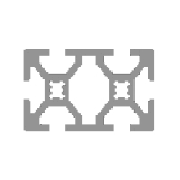
# Autodesk Inventor part: 20-2040
Saved by Autodesk Inventor 2021 (Build 250183000, 183)
## iProperties
IsCustomPart: 1
_CCFamilyDisplayName: 20-2040
_FrameMemberDoc: Frame Member File
_Version: 15.0.0
_GetPNFromCC: 1
Created: 2020-11-09
Part Number: 20-2040
Material: Generic
Document SubType Name: Modeling
Designer: Wes
Manufacturer: 8020
Standards Organization: 8020 Metric
Language: en-US
Size Designation: 20-2040
Categories: <MemberInstance><Categories><Category DisplayName="Structural Shapes" InternalName="089c4875-fa83-4c05-b084-43b9cc11f5ed" Mnemonic="GRDR"><CategoryParameter DisplayName="Mass per Length Unit" InternalName="0bb95a10-148f-4027-a459-38d7b056702a" Mnemonic="shpmass"/><CategoryParameter DisplayName="Section Area" InternalName="1ff91680-64b0-4202-b9a3-7fd3f94bba3b" Mnemonic="secarea"/><CategoryParameter DisplayName="Radius of Gyration (x)" InternalName="25778675-03e9-40c1-b6a8-4a9ed693320d" Mnemonic="gyrradx"/><CategoryParameter DisplayName="Torsional Rigidity Modulus" InternalName="26c1ec35-5026-4c63-ad0a-751cf684a536" Mnemonic="torrigmod"/><CategoryParameter DisplayName="Distance of the Center of Gravity X-X" InternalName="26c9bdb8-9c79-4b4f-a92e-8e197583c9c4" Mnemonic="grcendistX"/><CategoryParameter DisplayName="Legacy Member ID" InternalName="340afe4f-75d7-48d3-ab7d-943f3c3da468" Mnemonic="LegacyMemberID"/><CategoryParameter DisplayName="Base Length" InternalName="42e34263-8f20-4d0e-ad48-bf1385b87c24" Mnemonic="shplen"/><CategoryParameter DisplayName="Moment of Inertia (y)" InternalName="4b9f58ea-bced-460e-81ea-3d29ca5a49e3" Mnemonic="inermomy"/><CategoryParameter DisplayName="Moment of Inertia (x)" InternalName="4cd780bc-73d7-43ac-917a-579e5cbd684d" Mnemonic="inermomx"/><CategoryParameter DisplayName="Custom Base Point" InternalName="4f1d1b73-316d-484b-a3df-9cbabb16eb77" Mnemonic="shpBasePoint"/><CategoryParameter DisplayName="Shape Height" InternalName="50274e7d-5ac0-4796-92cb-c59e54983c67" Mnemonic="shpheig"/><CategoryParameter DisplayName="Section Module (y)" InternalName="59eaa5e9-d227-48dc-b6c1-6920f96e0f95" Mnemonic="secmody"/><CategoryParameter DisplayName="Section Designation" InternalName="5a64d034-428d-49c8-ba32-7619764de20f" Mnemonic="shpdes"/><CategoryParameter DisplayName="Section Module (x)" InternalName="72cfad18-cf51-4ed4-aaa7-c6b224f8419f" Mnemonic="secmodx"/><CategoryParameter DisplayName="Torsional Section Modulus" InternalName="7c55a8dc-8844-49f9-a867-cc677b30ec9a" Mnemonic="torsecmod"/><CategoryParameter DisplayName="Shape Width" InternalName="7c717d54-a18f-4666-b4d4-573cce22c62c" Mnemonic="shpwdth"/><CategoryParameter DisplayName="Second Shape Thickness" InternalName="9251a8e1-85fd-4e47-af99-afdb762317d9" Mnemonic="shpthick2"/><CategoryParameter DisplayName="FG Authored" InternalName="9c666724-f362-4ea7-ac62-f6a007de5c69" Mnemonic="shpFGAuto"/><CategoryParameter DisplayName="Distance of the Center of Gravity Y-Y" InternalName="bcc4fb17-7af4-436a-8f8c-d0aa3b0248c5" Mnemonic="grcendistY"/><CategoryParameter DisplayName="Radius of Gyration (y)" InternalName="bfa18ebe-1636-4dbe-8d42-b263e0b73184" Mnemonic="gyrrady"/><CategoryParameter DisplayName="Shape Thickness" InternalName="d109cf76-8eb4-42fc-9800-4409734adc67" Mnemonic="shpthick"/><CategoryParameter DisplayName="Coefficient of Shear Displacement" InternalName="de4c90c6-aaa8-468f-a335-6737b311b5d3" Mnemonic="shdispc"/><Category DisplayName="Other" InternalName="f02205ff-2390-476f-921c-0b3185f88e84" Mnemonic="OTHSHP"><CategoryParameter DisplayName="Moment of Inertia (y)" InternalName="044c654e-f649-48ac-84cc-650a29ae31ca" Mnemonic="inermomy"/><CategoryParameter DisplayName="Shape Thickness" InternalName="12b1a788-9233-48fd-a933-2df8ff42b15f" Mnemonic="shpthick"/><CategoryParameter DisplayName="Mass per Length Unit" InternalName="2fd289d6-9394-4d2d-97e6-6659d7d4551d" Mnemonic="shpmass"/><CategoryParameter DisplayName="Radius of Gyration (y)" InternalName="743e1dfe-1bba-408b-b985-cf752b207386" Mnemonic="gyrrady"/><CategoryParameter DisplayName="Section Module (y)" InternalName="88b8bff9-a616-4028-93d5-ed4f79680d13" Mnemonic="secmody"/><CategoryParameter DisplayName="Section Area" InternalName="c46ecdf8-b6eb-4db9-8b25-30258930c1e3" Mnemonic="secarea"/><CategoryParameter DisplayName="Section Module (x)" InternalName="cac70804-9d39-43bb-be17-56ea1f39a6c2" Mnemonic="secmodx"/><CategoryParameter DisplayName="Moment of Inertia (x)" InternalName="ec6737bc-264f-43ed-b0bd-f6d410c2718d" Mnemonic="inermomx"/><CategoryParameter DisplayName="Radius of Gyration (x)" InternalName="ee72c61e-565e-4fd6-b448-66e1e1abcb7e" Mnemonic="gyrradx"/><Category DisplayName="8020" InternalName="79851eee-1260-43d5-80eb-d25638456875" Mnemonic="8020"/></Category></Category><Category DisplayName="DataType" InternalName="23b78d0f-2648-40c6-8793-ca6db495c9e8" Mnemonic="DATATYPE"><CategoryParameter DisplayName="DisplayName" InternalName="05415f3d-3907-474b-a020-eb9d644f4cf3" Mnemonic="DISPLAYNAME"/><CategoryParameter DisplayName="Standard" InternalName="0c0a119c-1e12-4c84-803f-101930972f5e" Mnemonic="STANDARD"/><CategoryParameter DisplayName="Description" InternalName="13903e3d-64b1-4950-80da-f627842ea37f" Mnemonic="DESCRIPTION"/><CategoryParameter DisplayName="Designation" InternalName="2675968c-4ce5-49e0-a4f5-552d29089031" Mnemonic="DESIGNATION"/><CategoryParameter DisplayName="Default Row" InternalName="2af9ec52-faaa-4026-b378-f9fa4afca842" Mnemonic="DEFAULTROW"/><CategoryParameter DisplayName="Folder Name" InternalName="3f06958e-8713-4116-9be7-ed6184ecc97b" Mnemonic="FOLDERNAME"/><CategoryParameter DisplayName="Revision Guid" InternalName="45a75005-10b1-4dfc-8d6d-dfe629f0b93c" Mnemonic="REVISIONGUID"/><CategoryParameter DisplayName="FileName" InternalName="8b46a4cc-9585-4fed-90c3-899f57e09a73" Mnemonic="FILENAME"/><CategoryParameter DisplayName="StdsOrg" InternalName="8f5914e1-4693-403f-8ab5-d37768198c9d" Mnemonic="STDSORG"/><CategoryParameter DisplayName="Family Version" InternalName="914462f6-6e19-4b14-ba84-155b9680b1d0" Mnemonic="FAMILYREVISION"/><CategoryParameter DisplayName="Standard Revision" InternalName="91d5a463-65c2-4fde-b823-3b7fea5e8e17" Mnemonic="STANDARDREVISION"/><CategoryParameter DisplayName="Member Revision" InternalName="a65d44b9-392f-4f4f-857b-e4b3d54996fe" Mnemonic="MEMBERREVISION"/><CategoryParameter DisplayName="ClipFormat" InternalName="bc51e27b-3422-4e78-93ef-cec197ddf230" Mnemonic="CLIPFORMAT"/><CategoryParameter DisplayName="Manufacturer" InternalName="cd6c7a72-a28a-4e50-99a9-2c7f4e13e5ad" Mnemonic="MANUFACTURER"/><CategoryParameter DisplayName="InternalName" InternalName="cf1d0246-76d9-4b4a-8305-fa0409afb5c1" Mnemonic="INTERNALNAME"/><CategoryParameter DisplayName="IsMetric" InternalName="e2385c5b-1ea4-4823-96a8-8de651266ec3" Mnemonic="ISMETRIC"/><Category DisplayName="Part" InternalName="c0e0b642-3bcb-4cc8-9e80-f96d35c4afa4" Mnemonic="PART"><CategoryParameter DisplayName="Part Number" InternalName="016b6077-bfbe-49bd-92c9-d8d59c39c941" Mnemonic="PARTNUMBER"/><CategoryParameter DisplayName="Stock Number" InternalName="4dba7c1c-e26c-444e-836c-b08b433409a8" Mnemonic="STOCKNUMBER"/><CategoryParameter DisplayName="Material Key" InternalName="5c9a8adb-dd2b-4535-b97f-0a94a95fe41f" Mnemonic="MATERIALKEY"/><CategoryParameter DisplayName="Material" InternalName="818a152a-d3c3-49ca-80ee-df7d91421b8e" Mnemonic="MATERIAL"/></Category></Category></Categories><FamilyTemplate Id="20-2040"><FamilyTemplateParameters><FamilyTemplateParameter ObjectType="kModelParameterObject" ValueType="xs:double" Id="12" ObjectReferenceKey="Length"/><FamilyTemplateParameter ObjectType="kPartComponentDefinitionObject" ValueType="xs:string" Id="23" SubObjectId="Material"/><FamilyTemplateParameter ObjectType="kPropertyObject" ValueType="xs:string" Id="26" ObjectReferenceKey="{32853F0F-3444-11d1-9E93-0060B03C1CA6}" SubObjectId="5"/><FamilyTemplateParameter ObjectType="kPropertyObject" ValueType="xs:string" Id="27" ObjectReferenceKey="{32853F0F-3444-11d1-9E93-0060B03C1CA6}" SubObjectId="52"/></FamilyTemplateParameters></FamilyTemplate><CategoryParameterMap><ParamToTemplateMap><ParamToTemplate CategoryParameter="//CategoryParameter[@InternalName='cf1d0246-76d9-4b4a-8305-fa0409afb5c1']" ConstantValue="dee9908e-3317-4e3c-8f63-6ae0a76ae7af"/><ParamToTemplate CategoryParameter="//CategoryParameter[@InternalName='45a75005-10b1-4dfc-8d6d-dfe629f0b93c']" ConstantValue="6f377949-8875-44fd-a8fb-486841dd85e7"/><ParamToTemplate CategoryParameter="//CategoryParameter[@InternalName='3f06958e-8713-4116-9be7-ed6184ecc97b']" ConstantValue="20-2040"/><ParamToTemplate CategoryParameter="//CategoryParameter[@InternalName='8f5914e1-4693-403f-8ab5-d37768198c9d']" ConstantValue="8020 Metric"/><ParamToTemplate CategoryParameter="//CategoryParameter[@InternalName='0c0a119c-1e12-4c84-803f-101930972f5e']" TemplateParameter="18"/><ParamToTemplate CategoryParameter="//CategoryParameter[@InternalName='91d5a463-65c2-4fde-b823-3b7fea5e8e17']" TemplateParameter="19"/><ParamToTemplate CategoryParameter="//CategoryParameter[@InternalName='cd6c7a72-a28a-4e50-99a9-2c7f4e13e5ad']" ConstantValue="8020"/><ParamToTemplate CategoryParameter="//CategoryParameter[@InternalName='13903e3d-64b1-4950-80da-f627842ea37f']" TemplateParameter="22"/><ParamToTemplate CategoryParameter="//CategoryParameter[@InternalName='05415f3d-3907-474b-a020-eb9d644f4cf3']" ConstantValue="20-2040"/><ParamToTemplate CategoryParameter="//CategoryParameter[@InternalName='914462f6-6e19-4b14-ba84-155b9680b1d0']" ConstantValue="11"/><ParamToTemplate CategoryParameter="//CategoryParameter[@InternalName='bc51e27b-3422-4e78-93ef-cec197ddf230']" ConstantValue="CF_INVENTOR.STDPARTS"/><ParamToTemplate CategoryParameter="//CategoryParameter[@InternalName='e2385c5b-1ea4-4823-96a8-8de651266ec3']" ConstantValue="false"/><ParamToTemplate CategoryParameter="//CategoryParameter[@InternalName='2af9ec52-faaa-4026-b378-f9fa4afca842']" ConstantValue="1"/><ParamToTemplate CategoryParameter="//CategoryParameter[@InternalName='4f1d1b73-316d-484b-a3df-9cbabb16eb77']" ConstantValue="1"/><ParamToTemplate CategoryParameter="//CategoryParameter[@InternalName='9c666724-f362-4ea7-ac62-f6a007de5c69']" ConstantValue="1"/><ParamToTemplate CategoryParameter="//CategoryParameter[@InternalName='8b46a4cc-9585-4fed-90c3-899f57e09a73']" ConstantValue="20-2040"/><ParamToTemplate CategoryParameter="//CategoryParameter[@InternalName='a65d44b9-392f-4f4f-857b-e4b3d54996fe']" ConstantValue="4d23351e-7b41-4540-9885-5d219b5013c0"/><ParamToTemplate CategoryParameter="//CategoryParameter[@InternalName='a65d44b9-392f-4f4f-857b-e4b3d54996fe']" ConstantValue="4d23351e-7b41-4540-9885-5d219b5013c0"/><ParamToTemplate CategoryParameter="//CategoryParameter[@InternalName='2675968c-4ce5-49e0-a4f5-552d29089031']" TemplateParameter="27"/><ParamToTemplate CategoryParameter="//CategoryParameter[@InternalName='42e34263-8f20-4d0e-ad48-bf1385b87c24']" TemplateParameter="12"/><ParamToTemplate CategoryParameter="//CategoryParameter[@InternalName='818a152a-d3c3-49ca-80ee-df7d91421b8e']" TemplateParameter="23"/><ParamToTemplate CategoryParameter="//CategoryParameter[@InternalName='016b6077-bfbe-49bd-92c9-d8d59c39c941']" TemplateParameter="26"/></ParamToTemplateMap></CategoryParameterMap></MemberInstance>
Density: 1 g/cm^3
Appearance: Default
G_W: 1.575 in
G_H: 0.787 in
+B9D86D3A-4208-4660-9CD6-A881373FE610+CUTDETAIL2: Cut Angle 90.00 deg
+8888F257-0BC0-49C0-B35C-043E306DD604+CUTDETAIL1: Cut Angle 90.00 deg
G_L: 9.409 in
Author: Wes
Autodesk Inventor part; units mm, degrees
sketch "20-2040" plane through (0, 0, 0) normal (0, 0, 1) x (1, 0, 0)
  arc A0 (13.0994, 14.9012) -> (14.4203, 14.5318) centre (13.8638, 15.0883) ccw
  line L0 (14.4203, 14.5318) -> (14.5999, 14.7114)
  arc A1 (14.5999, 14.7114) -> (14.2305, 16.0323) centre (14.0434, 15.2679) ccw
  arc A2 (14.2305, 16.0323) -> (14.2305, 17.6403) centre (12.2954, 16.8363) ccw
  arc A3 (14.2305, 17.6403) -> (14.5999, 18.9612) centre (14.0434, 18.4047) ccw
  line L1 (14.5999, 18.9612) -> (14.4203, 19.1408)
  arc A4 (14.4203, 19.1408) -> (13.0994, 18.7714) centre (13.8638, 18.5843) ccw
  arc A5 (13.0994, 18.7714) -> (11.4914, 18.7714) centre (12.2954, 16.8363) ccw
  arc A6 (11.4914, 18.7714) -> (10.1705, 19.1408) centre (10.727, 18.5843) ccw
  line L2 (10.1705, 19.1408) -> (9.9909, 18.9612)
  arc A7 (9.9909, 18.9612) -> (10.3603, 17.6403) centre (10.5474, 18.4047) ccw
  arc A8 (10.3603, 17.6403) -> (10.3603, 16.0323) centre (12.2954, 16.8363) ccw
  arc A9 (10.3603, 16.0323) -> (9.9909, 14.7114) centre (10.5474, 15.2679) ccw
  line L3 (9.9909, 14.7114) -> (10.1705, 14.5318)
  arc A10 (10.1705, 14.5318) -> (11.4914, 14.9012) centre (10.727, 15.0883) ccw
  arc A11 (11.4914, 14.9012) -> (13.0994, 14.9012) centre (12.2954, 16.8363) ccw
  arc A12 (33.0994, 14.9012) -> (34.4203, 14.5318) centre (33.8638, 15.0883) ccw
  line L4 (34.4203, 14.5318) -> (34.5999, 14.7114)
  arc A13 (34.5999, 14.7114) -> (34.2305, 16.0323) centre (34.0434, 15.2679) ccw
  arc A14 (34.2305, 16.0323) -> (34.2305, 17.6403) centre (32.2954, 16.8363) ccw
  arc A15 (34.2305, 17.6403) -> (34.5999, 18.9612) centre (34.0434, 18.4047) ccw
  line L5 (34.5999, 18.9612) -> (34.4203, 19.1408)
  arc A16 (34.4203, 19.1408) -> (33.0994, 18.7714) centre (33.8638, 18.5843) ccw
  arc A17 (33.0994, 18.7714) -> (31.4914, 18.7714) centre (32.2954, 16.8363) ccw
  arc A18 (31.4914, 18.7714) -> (30.1705, 19.1408) centre (30.727, 18.5843) ccw
  line L6 (30.1705, 19.1408) -> (29.9909, 18.9612)
  arc A19 (29.9909, 18.9612) -> (30.3603, 17.6403) centre (30.5474, 18.4047) ccw
  arc A20 (30.3603, 17.6403) -> (30.3603, 16.0323) centre (32.2954, 16.8363) ccw
  arc A21 (30.3603, 16.0323) -> (29.9909, 14.7114) centre (30.5474, 15.2679) ccw
  line L7 (29.9909, 14.7114) -> (30.1705, 14.5318)
  arc A22 (30.1705, 14.5318) -> (31.4914, 14.9012) centre (30.727, 15.0883) ccw
  arc A23 (31.4914, 14.9012) -> (33.0994, 14.9012) centre (32.2954, 16.8363) ccw
  line L8 (6.4492, 9.9294) -> (9.5523, 13.0325)
  arc A24 (6.4492, 9.9294) -> (6.3004, 9.5702) centre (6.8084, 9.5702) ccw
  line L9 (6.3004, 8.8443) -> (6.3004, 9.5702)
  arc A25 (6.3004, 8.8443) -> (6.8084, 8.3363) centre (6.8084, 8.8443) ccw
  line L10 (9.1574, 8.3363) -> (6.8084, 8.3363)
  arc A26 (9.6654, 7.8283) -> (9.1574, 8.3363) centre (9.1574, 7.8283) ccw
  line L11 (9.6654, 7.3443) -> (9.6654, 7.8283)
  arc A27 (9.1574, 6.8363) -> (9.6654, 7.3443) centre (9.1574, 7.3443) ccw
  line L12 (3.7954, 6.8363) -> (9.1574, 6.8363)
  arc A28 (2.2954, 8.3363) -> (3.7954, 6.8363) centre (3.7954, 8.3363) ccw
  line L13 (2.2954, 13.6983) -> (2.2954, 8.3363)
  arc A29 (2.8034, 14.2063) -> (2.2954, 13.6983) centre (2.8034, 13.6983) ccw
  line L14 (3.2874, 14.2063) -> (2.8034, 14.2063)
  arc A30 (3.7954, 13.6983) -> (3.2874, 14.2063) centre (3.2874, 13.6983) ccw
  line L15 (3.7954, 11.3493) -> (3.7954, 13.6983)
  arc A31 (3.7954, 11.3493) -> (4.3034, 10.8413) centre (4.3034, 11.3493) ccw
  line L16 (5.0293, 10.8413) -> (4.3034, 10.8413)
  arc A32 (5.0293, 10.8413) -> (5.3885, 10.9901) centre (5.0293, 11.3493) ccw
  line L17 (8.4916, 14.0932) -> (5.3885, 10.9901)
  arc A33 (8.4916, 14.0932) -> (8.6404, 14.4524) centre (8.1324, 14.4524) ccw
  line L18 (8.6404, 19.2202) -> (8.6404, 14.4524)
  arc A34 (8.6404, 19.2202) -> (8.4916, 19.5794) centre (8.1324, 19.2202) ccw
  line L19 (5.3885, 22.6825) -> (8.4916, 19.5794)
  arc A35 (5.3885, 22.6825) -> (5.0293, 22.8313) centre (5.0293, 22.3233) ccw
  line L20 (4.3034, 22.8313) -> (5.0293, 22.8313)
  arc A36 (4.3034, 22.8313) -> (3.7954, 22.3233) centre (4.3034, 22.3233) ccw
  line L21 (3.7954, 19.9743) -> (3.7954, 22.3233)
  arc A37 (3.2874, 19.4663) -> (3.7954, 19.9743) centre (3.2874, 19.9743) ccw
  line L22 (2.8034, 19.4663) -> (3.2874, 19.4663)
  arc A38 (2.2954, 19.9743) -> (2.8034, 19.4663) centre (2.8034, 19.9743) ccw
  line L23 (2.2954, 25.3363) -> (2.2954, 19.9743)
  arc A39 (3.7954, 26.8363) -> (2.2954, 25.3363) centre (3.7954, 25.3363) ccw
  line L24 (9.1574, 26.8363) -> (3.7954, 26.8363)
  arc A40 (9.6654, 26.3283) -> (9.1574, 26.8363) centre (9.1574, 26.3283) ccw
  line L25 (9.6654, 25.8443) -> (9.6654, 26.3283)
  arc A41 (9.1574, 25.3363) -> (9.6654, 25.8443) centre (9.1574, 25.8443) ccw
  line L26 (6.8084, 25.3363) -> (9.1574, 25.3363)
  arc A42 (6.8084, 25.3363) -> (6.3004, 24.8283) centre (6.8084, 24.8283) ccw
  line L27 (6.3004, 24.1024) -> (6.3004, 24.8283)
  arc A43 (6.3004, 24.1024) -> (6.4492, 23.7432) centre (6.8084, 24.1024) ccw
  line L28 (9.5523, 20.6401) -> (6.4492, 23.7432)
  arc A44 (9.5523, 20.6401) -> (9.9115, 20.4913) centre (9.9115, 20.9993) ccw
  line L29 (14.6793, 20.4913) -> (9.9115, 20.4913)
  arc A45 (14.6793, 20.4913) -> (15.0385, 20.6401) centre (14.6793, 20.9993) ccw
  line L30 (18.1416, 23.7432) -> (15.0385, 20.6401)
  arc A46 (18.1416, 23.7432) -> (18.2904, 24.1024) centre (17.7824, 24.1024) ccw
  line L31 (18.2904, 24.8283) -> (18.2904, 24.1024)
  arc A47 (18.2904, 24.8283) -> (17.7824, 25.3363) centre (17.7824, 24.8283) ccw
  line L32 (15.4334, 25.3363) -> (17.7824, 25.3363)
  arc A48 (14.9254, 25.8443) -> (15.4334, 25.3363) centre (15.4334, 25.8443) ccw
  line L33 (14.9254, 26.3283) -> (14.9254, 25.8443)
  arc A49 (15.4334, 26.8363) -> (14.9254, 26.3283) centre (15.4334, 26.3283) ccw
  line L34 (29.1574, 26.8363) -> (15.4334, 26.8363)
  arc A50 (29.6654, 26.3283) -> (29.1574, 26.8363) centre (29.1574, 26.3283) ccw
  line L35 (29.6654, 25.8443) -> (29.6654, 26.3283)
  arc A51 (29.1574, 25.3363) -> (29.6654, 25.8443) centre (29.1574, 25.8443) ccw
  line L36 (26.8084, 25.3363) -> (29.1574, 25.3363)
  arc A52 (26.8084, 25.3363) -> (26.3004, 24.8283) centre (26.8084, 24.8283) ccw
  line L37 (26.3004, 24.1024) -> (26.3004, 24.8283)
  arc A53 (26.3004, 24.1024) -> (26.4492, 23.7432) centre (26.8084, 24.1024) ccw
  line L38 (29.5523, 20.6401) -> (26.4492, 23.7432)
  arc A54 (29.5523, 20.6401) -> (29.9115, 20.4913) centre (29.9115, 20.9993) ccw
  line L39 (34.6793, 20.4913) -> (29.9115, 20.4913)
  arc A55 (34.6793, 20.4913) -> (35.0385, 20.6401) centre (34.6793, 20.9993) ccw
  line L40 (38.1416, 23.7432) -> (35.0385, 20.6401)
  arc A56 (38.1416, 23.7432) -> (38.2904, 24.1024) centre (37.7824, 24.1024) ccw
  line L41 (38.2904, 24.8283) -> (38.2904, 24.1024)
  arc A57 (38.2904, 24.8283) -> (37.7824, 25.3363) centre (37.7824, 24.8283) ccw
  line L42 (35.4334, 25.3363) -> (37.7824, 25.3363)
  arc A58 (34.9254, 25.8443) -> (35.4334, 25.3363) centre (35.4334, 25.8443) ccw
  line L43 (34.9254, 26.3283) -> (34.9254, 25.8443)
  arc A59 (35.4334, 26.8363) -> (34.9254, 26.3283) centre (35.4334, 26.3283) ccw
  line L44 (40.7954, 26.8363) -> (35.4334, 26.8363)
  arc A60 (42.2954, 25.3363) -> (40.7954, 26.8363) centre (40.7954, 25.3363) ccw
  line L45 (42.2954, 19.9743) -> (42.2954, 25.3363)
  arc A61 (41.7874, 19.4663) -> (42.2954, 19.9743) centre (41.7874, 19.9743) ccw
  line L46 (41.3034, 19.4663) -> (41.7874, 19.4663)
  arc A62 (40.7954, 19.9743) -> (41.3034, 19.4663) centre (41.3034, 19.9743) ccw
  line L47 (40.7954, 22.3233) -> (40.7954, 19.9743)
  arc A63 (40.7954, 22.3233) -> (40.2874, 22.8313) centre (40.2874, 22.3233) ccw
  line L48 (39.5615, 22.8313) -> (40.2874, 22.8313)
  arc A64 (39.5615, 22.8313) -> (39.2023, 22.6825) centre (39.5615, 22.3233) ccw
  line L49 (36.0992, 19.5794) -> (39.2023, 22.6825)
  arc A65 (36.0992, 19.5794) -> (35.9504, 19.2202) centre (36.4584, 19.2202) ccw
  line L50 (35.9504, 14.4524) -> (35.9504, 19.2202)
  arc A66 (35.9504, 14.4524) -> (36.0992, 14.0932) centre (36.4584, 14.4524) ccw
  line L51 (39.2023, 10.9901) -> (36.0992, 14.0932)
  arc A67 (39.2023, 10.9901) -> (39.5615, 10.8413) centre (39.5615, 11.3493) ccw
  line L52 (40.2874, 10.8413) -> (39.5615, 10.8413)
  arc A68 (40.2874, 10.8413) -> (40.7954, 11.3493) centre (40.2874, 11.3493) ccw
  line L53 (40.7954, 13.6983) -> (40.7954, 11.3493)
  arc A69 (41.3034, 14.2063) -> (40.7954, 13.6983) centre (41.3034, 13.6983) ccw
  line L54 (41.7874, 14.2063) -> (41.3034, 14.2063)
  arc A70 (42.2954, 13.6983) -> (41.7874, 14.2063) centre (41.7874, 13.6983) ccw
  line L55 (42.2954, 8.3363) -> (42.2954, 13.6983)
  arc A71 (40.7954, 6.8363) -> (42.2954, 8.3363) centre (40.7954, 8.3363) ccw
  line L56 (35.4334, 6.8363) -> (40.7954, 6.8363)
  arc A72 (34.9254, 7.3443) -> (35.4334, 6.8363) centre (35.4334, 7.3443) ccw
  line L57 (34.9254, 7.8283) -> (34.9254, 7.3443)
  arc A73 (35.4334, 8.3363) -> (34.9254, 7.8283) centre (35.4334, 7.8283) ccw
  line L58 (37.7824, 8.3363) -> (35.4334, 8.3363)
  arc A74 (37.7824, 8.3363) -> (38.2904, 8.8443) centre (37.7824, 8.8443) ccw
  line L59 (38.2904, 9.5702) -> (38.2904, 8.8443)
  arc A75 (38.2904, 9.5702) -> (38.1416, 9.9294) centre (37.7824, 9.5702) ccw
  line L60 (35.0385, 13.0325) -> (38.1416, 9.9294)
  arc A76 (35.0385, 13.0325) -> (34.6793, 13.1813) centre (34.6793, 12.6733) ccw
  line L61 (29.9115, 13.1813) -> (34.6793, 13.1813)
  arc A77 (29.9115, 13.1813) -> (29.5523, 13.0325) centre (29.9115, 12.6733) ccw
  line L62 (26.4492, 9.9294) -> (29.5523, 13.0325)
  arc A78 (26.4492, 9.9294) -> (26.3004, 9.5702) centre (26.8084, 9.5702) ccw
  line L63 (26.3004, 8.8443) -> (26.3004, 9.5702)
  arc A79 (26.3004, 8.8443) -> (26.8084, 8.3363) centre (26.8084, 8.8443) ccw
  line L64 (29.1574, 8.3363) -> (26.8084, 8.3363)
  arc A80 (29.6654, 7.8283) -> (29.1574, 8.3363) centre (29.1574, 7.8283) ccw
  line L65 (29.6654, 7.3443) -> (29.6654, 7.8283)
  arc A81 (29.1574, 6.8363) -> (29.6654, 7.3443) centre (29.1574, 7.3443) ccw
  line L66 (15.4334, 6.8363) -> (29.1574, 6.8363)
  arc A82 (14.9254, 7.3443) -> (15.4334, 6.8363) centre (15.4334, 7.3443) ccw
  line L67 (14.9254, 7.8283) -> (14.9254, 7.3443)
  arc A83 (15.4334, 8.3363) -> (14.9254, 7.8283) centre (15.4334, 7.8283) ccw
  line L68 (17.7824, 8.3363) -> (15.4334, 8.3363)
  arc A84 (17.7824, 8.3363) -> (18.2904, 8.8443) centre (17.7824, 8.8443) ccw
  line L69 (18.2904, 9.5702) -> (18.2904, 8.8443)
  arc A85 (18.2904, 9.5702) -> (18.1416, 9.9294) centre (17.7824, 9.5702) ccw
  line L70 (15.0385, 13.0325) -> (18.1416, 9.9294)
  arc A86 (15.0385, 13.0325) -> (14.6793, 13.1813) centre (14.6793, 12.6733) ccw
  line L71 (9.9115, 13.1813) -> (14.6793, 13.1813)
  arc A87 (9.9115, 13.1813) -> (9.5523, 13.0325) centre (9.9115, 12.6733) ccw
  arc A88 (24.2924, 8.3363) -> (24.8004, 8.8443) centre (24.2924, 8.8443) ccw
  line L72 (24.8004, 8.8443) -> (24.8004, 10.1915)
  arc A89 (24.9492, 10.5508) -> (24.8004, 10.1915) centre (25.3084, 10.1915) ccw
  line L73 (24.9492, 10.5508) -> (28.4916, 14.0932)
  arc A90 (28.4916, 14.0932) -> (28.6404, 14.4524) centre (28.1324, 14.4524) ccw
  line L74 (28.6404, 14.4524) -> (28.6404, 19.2202)
  arc A91 (28.6404, 19.2202) -> (28.4916, 19.5794) centre (28.1324, 19.2202) ccw
  line L75 (28.4916, 19.5794) -> (24.9492, 23.1219)
  arc A92 (24.8004, 23.4811) -> (24.9492, 23.1219) centre (25.3084, 23.4811) ccw
  line L76 (24.8004, 23.4811) -> (24.8004, 24.8283)
  arc A93 (24.8004, 24.8283) -> (24.2924, 25.3363) centre (24.2924, 24.8283) ccw
  line L77 (24.2924, 25.3363) -> (20.2984, 25.3363)
  arc A94 (20.2984, 25.3363) -> (19.7904, 24.8283) centre (20.2984, 24.8283) ccw
  line L78 (19.7904, 24.8283) -> (19.7904, 23.4811)
  arc A95 (19.6416, 23.1219) -> (19.7904, 23.4811) centre (19.2824, 23.4811) ccw
  line L79 (19.6416, 23.1219) -> (16.0992, 19.5794)
  arc A96 (16.0992, 19.5794) -> (15.9504, 19.2202) centre (16.4584, 19.2202) ccw
  line L80 (15.9504, 19.2202) -> (15.9504, 14.4524)
  arc A97 (15.9504, 14.4524) -> (16.0992, 14.0932) centre (16.4584, 14.4524) ccw
  line L81 (16.0992, 14.0932) -> (19.6416, 10.5508)
  arc A98 (19.7904, 10.1915) -> (19.6416, 10.5508) centre (19.2824, 10.1915) ccw
  line L82 (19.7904, 10.1915) -> (19.7904, 8.8443)
  arc A99 (19.7904, 8.8443) -> (20.2984, 8.3363) centre (20.2984, 8.8443) ccw
  line L83 (20.2984, 8.3363) -> (24.2924, 8.3363)
ref_plane "Start Plane" through (0, 0, 20) normal (0, 0, 1) x (1, 0, 0)
ref_plane "End Plane" through (0, 0, 259) normal (0, 0, 1) x (1, 0, 0)
sketch "Sketch" plane through (0, 0, 0) normal (0, 0, 1) x (1, 0, 0)
  arc A0 (0.804, -1.9351) -> (2.1249, -2.3045) centre (1.5684, -1.748) ccw
  line L0 (2.1249, -2.3045) -> (2.3045, -2.1249)
  arc A1 (2.3045, -2.1249) -> (1.9351, -0.804) centre (1.748, -1.5684) ccw
  arc A2 (1.9351, -0.804) -> (1.9351, 0.804) centre (0, 0) ccw
  arc A3 (1.9351, 0.804) -> (2.3045, 2.1249) centre (1.748, 1.5684) ccw
  line L1 (2.3045, 2.1249) -> (2.1249, 2.3045)
  arc A4 (2.1249, 2.3045) -> (0.804, 1.9351) centre (1.5684, 1.748) ccw
  arc A5 (0.804, 1.9351) -> (-0.804, 1.9351) centre (0, 0) ccw
  arc A6 (-0.804, 1.9351) -> (-2.1249, 2.3045) centre (-1.5684, 1.748) ccw
  line L2 (-2.1249, 2.3045) -> (-2.3045, 2.1249)
  arc A7 (-2.3045, 2.1249) -> (-1.9351, 0.804) centre (-1.748, 1.5684) ccw
  arc A8 (-1.9351, 0.804) -> (-1.9351, -0.804) centre (0, 0) ccw
  arc A9 (-1.9351, -0.804) -> (-2.3045, -2.1249) centre (-1.748, -1.5684) ccw
  line L3 (-2.3045, -2.1249) -> (-2.1249, -2.3045)
  arc A10 (-2.1249, -2.3045) -> (-0.804, -1.9351) centre (-1.5684, -1.748) ccw
  arc A11 (-0.804, -1.9351) -> (0.804, -1.9351) centre (0, 0) ccw
  arc A12 (20.804, -1.9351) -> (22.1249, -2.3045) centre (21.5684, -1.748) ccw
  line L4 (22.1249, -2.3045) -> (22.3045, -2.1249)
  arc A13 (22.3045, -2.1249) -> (21.9351, -0.804) centre (21.748, -1.5684) ccw
  arc A14 (21.9351, -0.804) -> (21.9351, 0.804) centre (20, 0) ccw
  arc A15 (21.9351, 0.804) -> (22.3045, 2.1249) centre (21.748, 1.5684) ccw
  line L5 (22.3045, 2.1249) -> (22.1249, 2.3045)
  arc A16 (22.1249, 2.3045) -> (20.804, 1.9351) centre (21.5684, 1.748) ccw
  arc A17 (20.804, 1.9351) -> (19.196, 1.9351) centre (20, 0) ccw
  arc A18 (19.196, 1.9351) -> (17.8751, 2.3045) centre (18.4316, 1.748) ccw
  line L6 (17.8751, 2.3045) -> (17.6955, 2.1249)
  arc A19 (17.6955, 2.1249) -> (18.0649, 0.804) centre (18.252, 1.5684) ccw
  arc A20 (18.0649, 0.804) -> (18.0649, -0.804) centre (20, 0) ccw
  arc A21 (18.0649, -0.804) -> (17.6955, -2.1249) centre (18.252, -1.5684) ccw
  line L7 (17.6955, -2.1249) -> (17.8751, -2.3045)
  arc A22 (17.8751, -2.3045) -> (19.196, -1.9351) centre (18.4316, -1.748) ccw
  arc A23 (19.196, -1.9351) -> (20.804, -1.9351) centre (20, 0) ccw
  line L8 (-5.8462, -6.9069) -> (-2.7431, -3.8038)
  arc A24 (-5.8462, -6.9069) -> (-5.995, -7.2661) centre (-5.487, -7.2661) ccw
  line L9 (-5.995, -7.992) -> (-5.995, -7.2661)
  arc A25 (-5.995, -7.992) -> (-5.487, -8.5) centre (-5.487, -7.992) ccw
  line L10 (-3.138, -8.5) -> (-5.487, -8.5)
  arc A26 (-2.63, -9.008) -> (-3.138, -8.5) centre (-3.138, -9.008) ccw
  line L11 (-2.63, -9.492) -> (-2.63, -9.008)
  arc A27 (-3.138, -10) -> (-2.63, -9.492) centre (-3.138, -9.492) ccw
  line L12 (-8.5, -10) -> (-3.138, -10)
  arc A28 (-10, -8.5) -> (-8.5, -10) centre (-8.5, -8.5) ccw
  line L13 (-10, -3.138) -> (-10, -8.5)
  arc A29 (-9.492, -2.63) -> (-10, -3.138) centre (-9.492, -3.138) ccw
  line L14 (-9.008, -2.63) -> (-9.492, -2.63)
  arc A30 (-8.5, -3.138) -> (-9.008, -2.63) centre (-9.008, -3.138) ccw
  line L15 (-8.5, -5.487) -> (-8.5, -3.138)
  arc A31 (-8.5, -5.487) -> (-7.992, -5.995) centre (-7.992, -5.487) ccw
  line L16 (-7.2661, -5.995) -> (-7.992, -5.995)
  arc A32 (-7.2661, -5.995) -> (-6.9069, -5.8462) centre (-7.2661, -5.487) ccw
  line L17 (-3.8038, -2.7431) -> (-6.9069, -5.8462)
  arc A33 (-3.8038, -2.7431) -> (-3.655, -2.3839) centre (-4.163, -2.3839) ccw
  line L18 (-3.655, 2.3839) -> (-3.655, -2.3839)
  arc A34 (-3.655, 2.3839) -> (-3.8038, 2.7431) centre (-4.163, 2.3839) ccw
  line L19 (-6.9069, 5.8462) -> (-3.8038, 2.7431)
  arc A35 (-6.9069, 5.8462) -> (-7.2661, 5.995) centre (-7.2661, 5.487) ccw
  line L20 (-7.992, 5.995) -> (-7.2661, 5.995)
  arc A36 (-7.992, 5.995) -> (-8.5, 5.487) centre (-7.992, 5.487) ccw
  line L21 (-8.5, 3.138) -> (-8.5, 5.487)
  arc A37 (-9.008, 2.63) -> (-8.5, 3.138) centre (-9.008, 3.138) ccw
  line L22 (-9.492, 2.63) -> (-9.008, 2.63)
  arc A38 (-10, 3.138) -> (-9.492, 2.63) centre (-9.492, 3.138) ccw
  line L23 (-10, 8.5) -> (-10, 3.138)
  arc A39 (-8.5, 10) -> (-10, 8.5) centre (-8.5, 8.5) ccw
  line L24 (-3.138, 10) -> (-8.5, 10)
  arc A40 (-2.63, 9.492) -> (-3.138, 10) centre (-3.138, 9.492) ccw
  line L25 (-2.63, 9.008) -> (-2.63, 9.492)
  arc A41 (-3.138, 8.5) -> (-2.63, 9.008) centre (-3.138, 9.008) ccw
  line L26 (-5.487, 8.5) -> (-3.138, 8.5)
  arc A42 (-5.487, 8.5) -> (-5.995, 7.992) centre (-5.487, 7.992) ccw
  line L27 (-5.995, 7.2661) -> (-5.995, 7.992)
  arc A43 (-5.995, 7.2661) -> (-5.8462, 6.9069) centre (-5.487, 7.2661) ccw
  line L28 (-2.7431, 3.8038) -> (-5.8462, 6.9069)
  arc A44 (-2.7431, 3.8038) -> (-2.3839, 3.655) centre (-2.3839, 4.163) ccw
  line L29 (2.3839, 3.655) -> (-2.3839, 3.655)
  arc A45 (2.3839, 3.655) -> (2.7431, 3.8038) centre (2.3839, 4.163) ccw
  line L30 (5.8462, 6.9069) -> (2.7431, 3.8038)
  arc A46 (5.8462, 6.9069) -> (5.995, 7.2661) centre (5.487, 7.2661) ccw
  line L31 (5.995, 7.992) -> (5.995, 7.2661)
  arc A47 (5.995, 7.992) -> (5.487, 8.5) centre (5.487, 7.992) ccw
  line L32 (3.138, 8.5) -> (5.487, 8.5)
  arc A48 (2.63, 9.008) -> (3.138, 8.5) centre (3.138, 9.008) ccw
  line L33 (2.63, 9.492) -> (2.63, 9.008)
  arc A49 (3.138, 10) -> (2.63, 9.492) centre (3.138, 9.492) ccw
  line L34 (16.862, 10) -> (3.138, 10)
  arc A50 (17.37, 9.492) -> (16.862, 10) centre (16.862, 9.492) ccw
  line L35 (17.37, 9.008) -> (17.37, 9.492)
  arc A51 (16.862, 8.5) -> (17.37, 9.008) centre (16.862, 9.008) ccw
  line L36 (14.513, 8.5) -> (16.862, 8.5)
  arc A52 (14.513, 8.5) -> (14.005, 7.992) centre (14.513, 7.992) ccw
  line L37 (14.005, 7.2661) -> (14.005, 7.992)
  arc A53 (14.005, 7.2661) -> (14.1538, 6.9069) centre (14.513, 7.2661) ccw
  line L38 (17.2569, 3.8038) -> (14.1538, 6.9069)
  arc A54 (17.2569, 3.8038) -> (17.6161, 3.655) centre (17.6161, 4.163) ccw
  line L39 (22.3839, 3.655) -> (17.6161, 3.655)
  arc A55 (22.3839, 3.655) -> (22.7431, 3.8038) centre (22.3839, 4.163) ccw
  line L40 (25.8462, 6.9069) -> (22.7431, 3.8038)
  arc A56 (25.8462, 6.9069) -> (25.995, 7.2661) centre (25.487, 7.2661) ccw
  line L41 (25.995, 7.992) -> (25.995, 7.2661)
  arc A57 (25.995, 7.992) -> (25.487, 8.5) centre (25.487, 7.992) ccw
  line L42 (23.138, 8.5) -> (25.487, 8.5)
  arc A58 (22.63, 9.008) -> (23.138, 8.5) centre (23.138, 9.008) ccw
  line L43 (22.63, 9.492) -> (22.63, 9.008)
  arc A59 (23.138, 10) -> (22.63, 9.492) centre (23.138, 9.492) ccw
  line L44 (28.5, 10) -> (23.138, 10)
  arc A60 (30, 8.5) -> (28.5, 10) centre (28.5, 8.5) ccw
  line L45 (30, 3.138) -> (30, 8.5)
  arc A61 (29.492, 2.63) -> (30, 3.138) centre (29.492, 3.138) ccw
  line L46 (29.008, 2.63) -> (29.492, 2.63)
  arc A62 (28.5, 3.138) -> (29.008, 2.63) centre (29.008, 3.138) ccw
  line L47 (28.5, 5.487) -> (28.5, 3.138)
  arc A63 (28.5, 5.487) -> (27.992, 5.995) centre (27.992, 5.487) ccw
  line L48 (27.2661, 5.995) -> (27.992, 5.995)
  arc A64 (27.2661, 5.995) -> (26.9069, 5.8462) centre (27.2661, 5.487) ccw
  line L49 (23.8038, 2.7431) -> (26.9069, 5.8462)
  arc A65 (23.8038, 2.7431) -> (23.655, 2.3839) centre (24.163, 2.3839) ccw
  line L50 (23.655, -2.3839) -> (23.655, 2.3839)
  arc A66 (23.655, -2.3839) -> (23.8038, -2.7431) centre (24.163, -2.3839) ccw
  line L51 (26.9069, -5.8462) -> (23.8038, -2.7431)
  arc A67 (26.9069, -5.8462) -> (27.2661, -5.995) centre (27.2661, -5.487) ccw
  line L52 (27.992, -5.995) -> (27.2661, -5.995)
  arc A68 (27.992, -5.995) -> (28.5, -5.487) centre (27.992, -5.487) ccw
  line L53 (28.5, -3.138) -> (28.5, -5.487)
  arc A69 (29.008, -2.63) -> (28.5, -3.138) centre (29.008, -3.138) ccw
  line L54 (29.492, -2.63) -> (29.008, -2.63)
  arc A70 (30, -3.138) -> (29.492, -2.63) centre (29.492, -3.138) ccw
  line L55 (30, -8.5) -> (30, -3.138)
  arc A71 (28.5, -10) -> (30, -8.5) centre (28.5, -8.5) ccw
  line L56 (23.138, -10) -> (28.5, -10)
  arc A72 (22.63, -9.492) -> (23.138, -10) centre (23.138, -9.492) ccw
  line L57 (22.63, -9.008) -> (22.63, -9.492)
  arc A73 (23.138, -8.5) -> (22.63, -9.008) centre (23.138, -9.008) ccw
  line L58 (25.487, -8.5) -> (23.138, -8.5)
  arc A74 (25.487, -8.5) -> (25.995, -7.992) centre (25.487, -7.992) ccw
  line L59 (25.995, -7.2661) -> (25.995, -7.992)
  arc A75 (25.995, -7.2661) -> (25.8462, -6.9069) centre (25.487, -7.2661) ccw
  line L60 (22.7431, -3.8038) -> (25.8462, -6.9069)
  arc A76 (22.7431, -3.8038) -> (22.3839, -3.655) centre (22.3839, -4.163) ccw
  line L61 (17.6161, -3.655) -> (22.3839, -3.655)
  arc A77 (17.6161, -3.655) -> (17.2569, -3.8038) centre (17.6161, -4.163) ccw
  line L62 (14.1538, -6.9069) -> (17.2569, -3.8038)
  arc A78 (14.1538, -6.9069) -> (14.005, -7.2661) centre (14.513, -7.2661) ccw
  line L63 (14.005, -7.992) -> (14.005, -7.2661)
  arc A79 (14.005, -7.992) -> (14.513, -8.5) centre (14.513, -7.992) ccw
  line L64 (16.862, -8.5) -> (14.513, -8.5)
  arc A80 (17.37, -9.008) -> (16.862, -8.5) centre (16.862, -9.008) ccw
  line L65 (17.37, -9.492) -> (17.37, -9.008)
  arc A81 (16.862, -10) -> (17.37, -9.492) centre (16.862, -9.492) ccw
  line L66 (3.138, -10) -> (16.862, -10)
  arc A82 (2.63, -9.492) -> (3.138, -10) centre (3.138, -9.492) ccw
  line L67 (2.63, -9.008) -> (2.63, -9.492)
  arc A83 (3.138, -8.5) -> (2.63, -9.008) centre (3.138, -9.008) ccw
  line L68 (5.487, -8.5) -> (3.138, -8.5)
  arc A84 (5.487, -8.5) -> (5.995, -7.992) centre (5.487, -7.992) ccw
  line L69 (5.995, -7.2661) -> (5.995, -7.992)
  arc A85 (5.995, -7.2661) -> (5.8462, -6.9069) centre (5.487, -7.2661) ccw
  line L70 (2.7431, -3.8038) -> (5.8462, -6.9069)
  arc A86 (2.7431, -3.8038) -> (2.3839, -3.655) centre (2.3839, -4.163) ccw
  line L71 (-2.3839, -3.655) -> (2.3839, -3.655)
  arc A87 (-2.3839, -3.655) -> (-2.7431, -3.8038) centre (-2.3839, -4.163) ccw
  arc A88 (11.997, -8.5) -> (12.505, -7.992) centre (11.997, -7.992) ccw
  line L72 (12.505, -7.992) -> (12.505, -6.6448)
  arc A89 (12.6538, -6.2856) -> (12.505, -6.6448) centre (13.013, -6.6448) ccw
  line L73 (12.6538, -6.2856) -> (16.1962, -2.7431)
  arc A90 (16.1962, -2.7431) -> (16.345, -2.3839) centre (15.837, -2.3839) ccw
  line L74 (16.345, -2.3839) -> (16.345, 2.3839)
  arc A91 (16.345, 2.3839) -> (16.1962, 2.7431) centre (15.837, 2.3839) ccw
  line L75 (16.1962, 2.7431) -> (12.6538, 6.2856)
  arc A92 (12.505, 6.6448) -> (12.6538, 6.2856) centre (13.013, 6.6448) ccw
  line L76 (12.505, 6.6448) -> (12.505, 7.992)
  arc A93 (12.505, 7.992) -> (11.997, 8.5) centre (11.997, 7.992) ccw
  line L77 (11.997, 8.5) -> (8.003, 8.5)
  arc A94 (8.003, 8.5) -> (7.495, 7.992) centre (8.003, 7.992) ccw
  line L78 (7.495, 7.992) -> (7.495, 6.6448)
  arc A95 (7.3462, 6.2856) -> (7.495, 6.6448) centre (6.987, 6.6448) ccw
  line L79 (7.3462, 6.2856) -> (3.8038, 2.7431)
  arc A96 (3.8038, 2.7431) -> (3.655, 2.3839) centre (4.163, 2.3839) ccw
  line L80 (3.655, 2.3839) -> (3.655, -2.3839)
  arc A97 (3.655, -2.3839) -> (3.8038, -2.7431) centre (4.163, -2.3839) ccw
  line L81 (3.8038, -2.7431) -> (7.3462, -6.2856)
  arc A98 (7.495, -6.6448) -> (7.3462, -6.2856) centre (6.987, -6.6448) ccw
  line L82 (7.495, -6.6448) -> (7.495, -7.992)
  arc A99 (7.495, -7.992) -> (8.003, -8.5) centre (8.003, -7.992) ccw
  line L83 (8.003, -8.5) -> (11.997, -8.5)
  point P0 (0, 0)
  constraints: 1 other
extrude "Body" add sketch "Sketch" along normal up to surface (239 mm away) from surface at 20
sketch "Sketch2" plane through (0, 0, 0) normal (0, 0, 1) x (1, 0, 0)
  line L0 (0, 0) -> (10, 0)
ref_plane "Work Plane3" through (0, 0, 0) normal (0, -1, 0) x (1, 0, 0)
sketch "Sketch3" plane through (0, 0, 0) normal (0, -1, 0) x (1, 0, 0)
  line L0 (-2, 20) -> (12, 20)
  line L1 (-2, 259) -> (12, 259)
  dimension "d7" = 239
  measures "d7" distance between parallel lines of L0 L1
ref_plane "Work Plane5" through (-269.4, 3.138, 259) normal (0, 0, 1) x (1, 0, 0)
split "Split2" plane through (-269.4, 3.138, 259) removes the side toward (0, 0, 1)
ref_plane "Work Plane6" through (-269.4, 8.5, 20) normal (0, 0, -1) x (-1, 0, 0)
split "Split3" plane through (-269.4, 8.5, 20) removes the side toward (0, 0, -1)
equation "\"G_OFFSET_START\" = -20"
equation "\"G_OFFSET_END\" = -20"
equation "\"d2\" = -G_OFFSET_START"
equation "\"d3\" = Length + G_OFFSET_END"
equation "\"G_L\" = d7"
equation "\"Length\" = 279"
body "Solid1"
